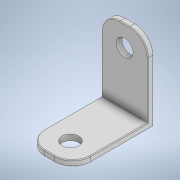
# Autodesk Inventor part: Right Angle
Saved by Autodesk Inventor 2022.1 (Build 261234020, 234B)
## iProperties
Created: 2023-10-09
Part Number: Right Angle
Material: Generic
Document SubType Name: Modeling
Designer: luke.macenski3281
Density: 1 g/cm^3
Appearance: Default
Author: luke.macenski3281
Autodesk Inventor part; units mm, degrees
ref_plane "YZ Plane" through (0, 0, 0) normal (1, 0, 0) x (0, 1, 0)
ref_plane "XZ Plane" through (0, 0, 0) normal (0, 1, 0) x (-1, 0, 0)
ref_plane "XY Plane" through (0, 0, 0) normal (0, 0, 1) x (1, 0, 0)
sketch "Sketch1" plane through (0, 0, 0) normal (0, 1, 0) x (-1, 0, 0)
  point P0 (0, 0)
sketch "Sketch2" plane through (0, 0, 0) normal (0, 1, 0) x (-1, 0, 0)
  line L0 (0, 0) -> (-16.129, 0)
  line L1 (-16.129, 0) -> (-16.129, 28.194)
  line L2 (-16.129, 28.194) -> (0, 28.194)
  line L3 (0, 28.194) -> (0, 0)
  circle A0 centre (-8.0645, 20.9296) radius 2.9464
  point P0 (-8.0645, 28.194)
  dimension "d0" = 16.129
  dimension "d1" = 28.194
  dimension "d3" = 5.8928
  dimension "d4" = 7.2644
  constraints: 8 end point, 2 parallel, 1 centre point, 1 horizontal, 1 midpoint, 1 perpendicular
  measures "d0" distance of L1.end L2.end
  measures "d1" distance from line of point (-8.065, 28.194) L0
  measures "d3" diameter of A0
  measures "d4" distance of point (-8.065, 28.194) A0.centre
extrude "Extrusion1" add sketch "Sketch2" along normal blind 2.0066
sketch "Sketch3" plane through (0, 0, 0) normal (0, -1, 0) x (1, 0, 0)
  line L0 (16.129, 0) -> (0, 0) projected
  line L1 (0, 0) -> (16.129, 0)
  line L2 (16.129, 0) -> (16.129, 2.0066)
  line L3 (16.129, 2.0066) -> (0, 2.0066)
  line L4 (0, 2.0066) -> (0, 0)
  point P0 (8.0645, 2.0066)
  dimension "d7" = 2.0066
  constraints: 8 end point, 2 parallel, 1 horizontal, 1 midpoint, 1 perpendicular
  measures "d7" distance from line of L0 point (8.065, 2.007)
extrude "Extrusion2" add sketch "Sketch3" against normal blind 27.94
fillet "Fillet1" radius 6.35 2 edges at (16.129, 1.0033, 28.194) (0, 1.0033, 28.194)
sketch "Sketch4" plane through (0, 2.0066, 2.0066) normal (0, 0, 1) x (1, 0, 0)
  circle A0 centre (8.0645, 18.669) radius 2.9464
  line L0 (0, 25.9334) -> (16.129, 25.9334) projected
  point P0 (0, -2.0066)
  point P1 (8.0645, 25.9334)
  dimension "d11" = 5.8928
  dimension "d12" = 7.2644
  constraints: 1 centre point, 1 midpoint
  measures "d11" diameter of A0
  measures "d12" distance of point (8.065, 25.933) A0.centre
fillet "Fillet2" radius 6.35 2 edges at (0, 27.94, 1.0033) (16.129, 27.94, 1.0033)
extrude "Extrusion3" cut sketch "Sketch4" against normal blind 2.0066
fillet "Fillet3" radius 0.254 20 edges at (14.2691, 2.0066, 26.3341) (8.0645, 2.0066, 28.194) (1.8599, 2.0066, 26.3341) (0, 2.0066, 11.9253) (16.129, 2.0066, 11.9253) (14.2691, 0, 26.3341) (8.0645, 0, 28.194) (1.8599, 0, 26.3341) (0, 0, 10.922) (16.129, 0, 10.922) (14.2691, 26.0801, 2.0066) (8.0645, 27.94, 2.0066) (1.8599, 26.0801, 2.0066) (0, 11.7983, 2.0066) (16.129, 11.7983, 2.0066) (14.2691, 26.0801, 0) (8.0645, 27.94, 0) (1.8599, 26.0801, 0) (0, 10.795, 0) (16.129, 10.795, 0)
body "Solid1"
